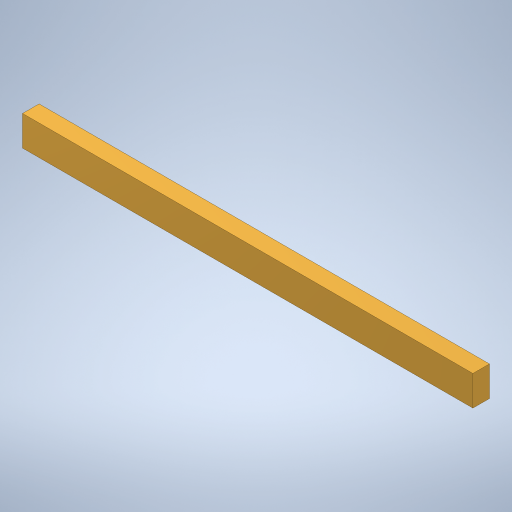
# Autodesk Inventor part: pen3_barra
Saved by Autodesk Inventor 2024.2 (Build 282272000, 272)
## iProperties
Created: 2024-04-15
Part Number: pen3_barra
Material: Brass, Soft Yellow
Document SubType Name: Modeling
Designer: 082220022
Density: 8.47 g/cm^3
Appearance: Brass - Satin
Author: 082220022
Autodesk Inventor part; units mm, degrees
ref_plane "YZ Plane" through (0, 0, 0) normal (1, 0, 0) x (0, 1, 0)
ref_plane "XZ Plane" through (0, 0, 0) normal (0, 1, 0) x (-1, 0, 0)
ref_plane "XY Plane" through (0, 0, 0) normal (0, 0, 1) x (1, 0, 0)
sketch "Sketch1" plane through (0, 0, 0) normal (0, 0, 1) x (1, 0, 0)
  line L0 (-3.1291, 5.172) -> (11.8709, 5.172)
  line L1 (11.8709, 5.172) -> (11.8709, 4.172)
  line L2 (11.8709, 4.172) -> (-3.1291, 4.172)
  line L3 (-3.1291, 4.172) -> (-3.1291, 5.172)
  point P0 (0, 0)
  dimension "d0" = 15
  dimension "d1" = 1
  constraints: 8 end point, 2 parallel, 1 horizontal, 1 perpendicular
  measures "d0" distance of L1.end L2.end
  measures "d1" distance of L0.end L1.end
extrude "Extrusion1" add sketch "Sketch1" along normal mid plane 0.55
body "Solid1"
